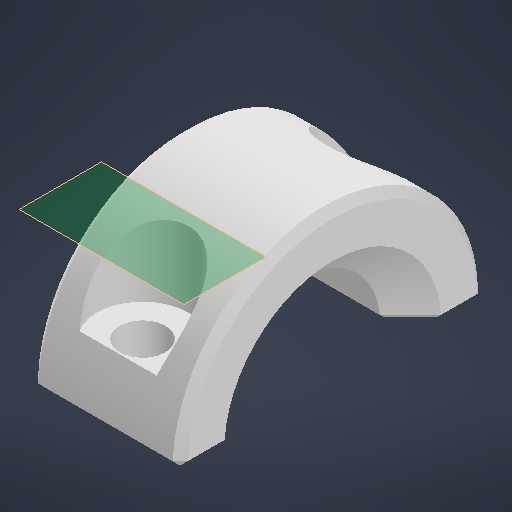
# Autodesk Inventor part: ForkTop
Saved by Autodesk Inventor 2026.3 (Build 303398000, 398)
## iProperties
Created: 2026-05-02
Part Number: ForkTop
Material: Generic
Document SubType Name: Modeling
Designer: frede
Density: 1 g/cm^3
Appearance: Default
Author: frede
Autodesk Inventor part; units mm, degrees
ref_plane "YZ Plane" through (0, 0, 0) normal (1, 0, 0) x (0, 1, 0)
ref_plane "XZ Plane" through (0, 0, 0) normal (0, 1, 0) x (-1, 0, 0)
ref_plane "XY Plane" through (0, 0, 0) normal (0, 0, 1) x (1, 0, 0)
sketch "Sketch1" plane through (0, 0, 0) normal (1, 0, 0) x (0, 1, 0)
  arc A0 (0, -5.1) -> (0, 5.1) centre (0, 0) ccw
  arc A1 (0, -10) -> (0, 10) centre (0, 0) ccw
  line L0 (0, 10) -> (0, 5.1)
  line L1 (0, -5.1) -> (0, -10)
  dimension "d0" = 10.2
  dimension "d1" = 20
  constraints: 4 end point, 4 point on circle, 2 centre point, 2 coincident, 2 point on line, 1 vertical
  measures "d0" diameter of A0
  measures "d1" diameter of A1
extrude "Extrusion1" add sketch "Sketch1" along normal blind 9.8
sketch "Sketch2" plane through (0, 0, 5.1) normal (0, -1, 0) x (1, 0, 0)
  line L0 (0, 4.9) -> (0, 0) projected
  line L1 (0, 0) -> (9.8, 0) projected
  line L2 (0, 4.9) -> (9.8, 0)
  line L3 (0, -10.2) -> (9.8, -10.2) projected
  line L4 (0, -15.1) -> (9.8, -15.1) projected
  line L5 (0, -10.2) -> (9.8, -15.1)
  point P0 (0, -5.1)
  point P1 (4.9, 2.45)
  point P2 (4.9, -12.65)
  constraints: 4 end point, 2 midpoint
hole "Hole1" at (4.9, 0, 7.55) at (4.9, 0, -7.55) direction (0, 1, 0) diameter 3 end through all countersink diameter 3.5 countersink angle 90
ref_plane "Work Plane1" through (0, 10, 5.1) normal (0, -1, 0) x (1, 0, 0)
sketch "Sketch3" plane through (0, 10, 5.1) normal (0, -1, 0) x (1, 0, 0)
  circle A0 centre (4.9, -12.65) radius 1.5 projected
  circle A1 centre (4.9, -12.65) radius 3
  circle A2 centre (4.9, 2.45) radius 1.5 projected
  circle A3 centre (4.9, 2.45) radius 3
  point P0 (0, -5.1)
  dimension "d12" = 6
  dimension "d13" = 6
  constraints: 2 centre point, 2 coincident
  measures "d12" diameter of A1
  measures "d13" diameter of A3
extrude "Extrusion2" cut sketch "Sketch3" along normal blind 6 contours A0 | A1 | A2 | A3
chamfer "Chamfer1" distance 2 angle 45 2 edges at (9.8, 5.1, 0) (0, 5.1, 0)
chamfer "Chamfer2" distance 0.5 angle 45 14 edges at (9.8, 10, 0) (9.8, 0, 8.55) (4.9, 0, 10) (0, 10, 0) (9.8, 0, -8.55) (8.8, 0, -6.1) (4.9, 0, -5.1) (0, 0, 8.55) (1, 0, 6.1) (4.9, 0, 5.1) (8.8, 0, 6.1) (1, 0, -6.1) (0, 0, -8.55) (4.9, 0, -10)
body "Solid1"
